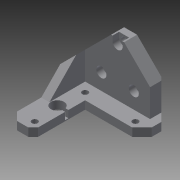
# Autodesk Inventor part: z-axis-bottom
Saved by Autodesk Inventor 2015 SP2 (Build 190223200, 223)
## iProperties
Created: 2015-05-29
Part Number: z-axis-bottom
Material: Generic
Document SubType Name: Modeling
Designer: X
Density: 1 g/cm^3
Appearance: Default
Author: X
Autodesk Inventor part; units mm, degrees
ref_plane "YZ Plane" through (0, 0, 0) normal (1, 0, 0) x (0, 1, 0)
ref_plane "XZ Plane" through (0, 0, 0) normal (0, 1, 0) x (-1, 0, 0)
ref_plane "XY Plane" through (0, 0, 0) normal (0, 0, 1) x (1, 0, 0)
sketch "Sketch2" plane through (0, 0, 0) normal (0, 0, 1) x (1, 0, 0)
  line L0 (0, 0) -> (50, 0)
  line L1 (50, 0) -> (50, 50)
  line L2 (50, 50) -> (0, 50)
  line L3 (0, 50) -> (0, 0)
  dimension "d0" = 50
  dimension "d1" = 50
  constraints: 8 end point, 2 parallel, 1 horizontal, 1 perpendicular
  measures "d0" distance of L2.end L0.start
  measures "d1" distance of L0.start L0.end
extrude "Extrusion1" add sketch "Sketch2" along normal blind 38
sketch "Sketch3" plane through (0, 0, 38) normal (0, 0, 1) x (1, 0, 0)
  line L0 (50, 0) -> (15, 0)
  line L1 (15, 0) -> (15, 32)
  line L2 (15, 32) -> (50, 32)
  line L3 (50, 32) -> (50, 0)
  line L4 (0, 50) -> (0, 0) projected
  line L5 (50, 50) -> (0, 50) projected
  dimension "d4" = 15
  dimension "d5" = 18
  constraints: 8 end point, 2 parallel, 1 horizontal, 1 perpendicular
  measures "d4" distance between parallel lines of L4 L1
  measures "d5" distance between parallel lines of L5 L2
extrude "Extrusion2" cut sketch "Sketch3" against normal through all
sketch "Sketch4" plane through (0, 0, 38) normal (0, 0, 1) x (1, 0, 0)
  line L0 (50, 32) -> (50, 50) projected
  line L1 (0, 0) -> (15, 0) projected
  line L2 (50, 42) -> (5, 42)
  line L3 (50, 50) -> (0, 50) projected
  line L4 (5, 42) -> (5, 0)
  line L5 (0, 50) -> (0, 0) projected
  line L6 (5, 0) -> (50, 0)
  line L7 (50, 0) -> (50, 42)
  dimension "d8" = 8
  dimension "d9" = 5
  constraints: 8 end point, 2 horizontal, 2 point on line, 1 perpendicular, 1 vertical
  measures "d8" distance between parallel lines of L2 L3
  measures "d9" distance between parallel lines of L5 L4
extrude "Extrusion3" cut sketch "Sketch4" against normal blind 33 contours L7 L6 L1 L4 L2 L0
sketch "Sketch6" plane through (0, 0, 0) normal (0, 1, 0) x (-1, 0, 0)
  line L0 (0, 17) -> (-21, 38)
  line L1 (-21, 38) -> (-29, 38)
  line L2 (0, 0) -> (0, 38) projected
  line L3 (-29, 38) -> (-45, 22)
  line L4 (-5, 38) -> (-50, 38) projected
  line L5 (-45, 22) -> (-45, 5)
  line L6 (-45, 5) -> (-50, 5)
  line L7 (-50, 5) -> (-50, 0)
  line L8 (-50, 0) -> (0, 0)
  line L9 (0, 17) -> (0, 0)
  dimension "d12" = 8
  dimension "d13" = 5
  dimension "d14" = 5
  dimension "d15" = 135
  dimension "d16" = 135
  dimension "d17" = 17
  constraints: 16 end point, 5 perpendicular, 1 collinear, 1 point on line, 1 vertical
  measures "d12" distance of L0.end L1.end
  measures "d13" distance of L5.end L6.end
  measures "d14" distance of L6.end L7.end
  measures "d15" angle of L5 L3
  measures "d16" angle of L2 L0
  measures "d17" distance of L3.end L5.end
extrude "Extrusion4" cut sketch "Sketch6" along normal through all keep common part
sketch "Sketch8" plane through (0, 0, 0) normal (1, 0, 0) x (0, 1, 0)
  line L0 (42, 38) -> (42, 22)
  line L1 (42, 22) -> (36.5, 22)
  line L2 (36.5, 22) -> (20, 5)
  line L3 (20, 5) -> (0, 5)
  line L4 (0, 5) -> (0, 38)
  line L5 (0, 38) -> (42, 38)
  line L6 (42, 22) -> (42, 38) projected
  line L7 (42, 38) -> (50, 38) projected
  line L8 (0, 22) -> (42, 22) projected
  line L9 (0, 0) -> (0, 17) projected
  dimension "d20" = 17
  dimension "d21" = 5.5
  dimension "d22" = 20
  constraints: 12 end point, 4 collinear, 2 parallel, 2 perpendicular, 1 vertical
  measures "d20" distance between parallel lines of L3 L1
  measures "d21" distance of L0.end L1.end
  measures "d22" distance of L2.end L3.end
extrude "Extrusion5" cut sketch "Sketch8" along normal through all
chamfer "Chamfer1" distance 5 distance2 5 1 edges at (0, 0, 2.5) measured on face at (0, 33.8824, 7.3333)
chamfer "Chamfer2" distance 3 distance2 3 1 edges at (15, 0, 2.5) measured on face at (8.3333, 0, 1.6667)
chamfer "Chamfer3" distance 6 distance2 6 1 edges at (50, 32, 2.5) measured on face at (50, 44, 3.3333)
chamfer "Chamfer4" distance 6 distance2 6 1 edges at (50, 50, 2.5) measured on face at (50, 46, 3.3333)
sketch "Sketch9" plane through (21, 42, 38) normal (0, -1, 0) x (1, 0, 0)
  line L0 (-6, -23) -> (14, -23) construction
  line L1 (23, -38) -> (-6, -38) construction
  line L2 (4, 0) -> (4, -38) construction
  line L3 (0, 0) -> (8, 0) construction
  point P0 (-21, -38)
  point P1 (4, -3)
  dimension "d37" = 20
  dimension "d38" = 10
  dimension "d39" = 20
  dimension "d40" = 3
  constraints: 4 end point, 2 point on line, 1 horizontal, 1 midpoint, 1 parallel, 1 perpendicular
  measures "d37" distance of L0.end L0.start
  measures "d38" horizontal distance of L0.end point (4, -3)
  measures "d39" distance from line of L0 point (4, -3)
  measures "d40" distance from line of L3 point (4, -3)
hole "Hole1" at (25, 42, 35) at (15, 42, 15) at (35, 42, 15) direction (0, 1, 0) diameter 3.6 end through all counterbore diameter 6.2 counterbore depth 4
sketch "Sketch10" plane through (0, 0, 5) normal (0, 0, 1) x (1, 0, 0)
  line L0 (10.8, 36.2) -> (10.8, 5.2) construction
  line L1 (10.8, 36.2) -> (41.8, 36.2) construction
  line L2 (44, 32) -> (15, 32) construction
  line L3 (15, 32) -> (15, 3) construction
  point P0 (0, 0)
  dimension "d48" = 4.2
  dimension "d49" = 4.2
  dimension "d50" = 31
  dimension "d51" = 31
  constraints: 4 end point, 1 horizontal, 1 vertical
  measures "d48" distance between parallel lines of L2 L1
  measures "d49" distance between parallel lines of L3 L0
  measures "d50" distance of L0.end L0.start
  measures "d51" distance of L1.end L0.start
hole "Hole2" at (41.8, 36.2, 5) at (10.8, 36.2, 5) at (10.8, 5.2, 5) direction (0, 0, -1) diameter 3.6 end through all
sketch "Sketch11" plane through (0, 0, 5) normal (0, 0, 1) x (1, 0, 0)
  line L0 (15, 32) -> (15, 3) projected
  line L1 (12, 0) -> (5, 0) projected
  line L2 (5, 36.5) -> (5, 20) projected
  point P0 (0, 0)
  point P1 (9.3, 20.7)
  dimension "d60" = 20.7
  dimension "d77" = 4.3
  measures "d60" distance from line of L1 point (9.3, 20.7)
  measures "d77" distance from line of point (9.3, 20.7) L2
hole "Hole3" at (9.3, 20.7, 5) direction (0, 0, -1) diameter 8 end through all
sketch "Sketch12" plane through (15, 32, 5) normal (1, 0, 0) x (0, 0, -1)
  line L0 (0, -15.3) -> (0, -7.3) projected
  line L1 (4.4, -12.3) -> (0, -12.3)
  line L2 (0, -12.3) -> (0, -10.3)
  line L3 (0, -10.3) -> (4.4, -10.3)
  line L4 (4.4, -10.3) -> (4.4, -12.3)
  line L5 (4.4, -12.3) -> (0, -10.3) construction
  line L6 (0, -12.3) -> (4.4, -10.3) construction
  line L7 (0, -32) -> (5, -32) projected
  line L8 (5, -7.3) -> (5, -15.3) projected
  point P0 (2.2, -11.3)
  dimension "d68" = 20.7
  dimension "d69" = 0.6
  dimension "d70" = 2
  constraints: 12 end point, 2 midpoint, 2 parallel, 1 horizontal, 1 perpendicular, 1 point on line
  measures "d68" distance from line of L7 point (2.2, -11.3)
  measures "d69" distance between parallel lines of L8 L4
  measures "d70" distance between parallel lines of L3 L1
extrude "Extrusion6" cut sketch "Sketch12" against normal up to surface
sketch "Sketch13" plane through (0, 0, 38) normal (0, 0, 1) x (1, 0, 0)
  line L0 (44, 50) -> (0, 50) construction
  line L1 (25, 50) -> (25, 42) construction
  line L2 (5, 42) -> (45, 42) construction
  line L3 (21.9, 42) -> (28.1, 42)
  line L4 (28.1, 42) -> (28.1, 46)
  line L5 (28.1, 46) -> (21.9, 46)
  line L6 (21.9, 46) -> (21.9, 42)
  line L7 (21.9, 42) -> (28.1, 46) construction
  line L8 (28.1, 42) -> (21.9, 46) construction
  line L9 (29, 50) -> (21, 50) projected
  point P0 (0, 0)
  point P1 (25, 44)
  point P2 (25, 50)
  dimension "d73" = 6.2
  dimension "d74" = 4
  constraints: 14 end point, 4 midpoint, 3 point on line, 2 parallel, 1 collinear, 1 horizontal, 1 perpendicular
  measures "d73" distance of L4.end L5.end
  measures "d74" distance of L3.end L4.end
extrude "Extrusion7" cut sketch "Sketch13" against normal up to surface
equation "\"d38\" = 0.5 * d37"
equation "\"d68\" = d60"
equation "\"d73\" = d43"
equation "\"d43\" = 6.2"
body "Solid1"
